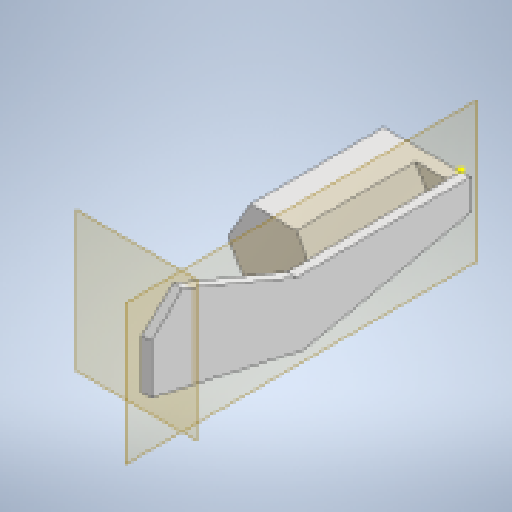
# Autodesk Inventor part: ArmSolenoidBoundingBoc
Saved by Autodesk Inventor 2023 (Build 270158000, 158)
## iProperties
Created: 2023-03-30
Part Number: ArmSolenoidBoundingBoc
Material: Generic
Document SubType Name: Modeling
Designer: LattePanda
Density: 1 g/cm^3
Appearance: Default
Author: LattePanda
Autodesk Inventor part; units mm, degrees
ref_plane "XZ Plane" through (0, 0, 0) normal (0, 1, 0) x (-1, 0, 0)
sketch "Sketch1" plane through (0, 0, 0) normal (1, 0, 0) x (0, 1, 0)
  line L0 (-24.1055, -88.5873) -> (-15.6118, -88.5873) construction
  line L1 (-20.9777, -35.0252) -> (-12.3846, 2.8126) construction
  line L2 (-11.1876, -82.4913) -> (-20.9871, -36.3884) construction
  line L3 (-10.1392, 12.7) -> (5.4091, 12.7)
  line L4 (5.4091, 12.7) -> (14.913, 2.8103)
  line L5 (14.913, 2.8103) -> (-0.1161, -33.4438)
  line L6 (-0.1161, -33.4438) -> (-0.1161, -88.5873)
  line L7 (-0.1161, -88.5873) -> (-9.8919, -88.5873)
  line L8 (-9.8919, -88.5873) -> (-21.1322, -35.7057)
  line L9 (-21.1322, -35.7057) -> (-10.1392, 12.7)
  line L10 (-0.1161, -27.3073) -> (-0.1161, -82.4913) construction
  arc A0 (9.8983, -7.957) -> (-12.3846, 2.8126) centre (0, 0) ccw construction
  point P0 (0, 0)
  constraints: 14 end point, 4 collinear, 3 tangent, 1 horizontal, 1 parallel
ref_plane "Work Plane1" through (3.048, -55.7199, -88.0008) normal (1, 0, 0) x (0, 0.7407454, 0.6717859)
extrude "Extrusion1" add sketch "Sketch1" along normal up to surface (3.048 mm away)
ref_plane "Work Plane2" through (86.0885, -0.1204, -88.5873) normal (0, 0, -1) x (0, -1, 0)
sketch "Sketch3" plane through (86.0885, -0.1204, -88.5873) normal (0, 0, -1) x (0, -1, 0)
  circle A0 centre (12.6956, 103.4693) radius 9.525 projected
  line L0 (12.6956, 89.0216) -> (0.1835, 96.2455)
  line L1 (0.1835, 96.2455) -> (0.1835, 110.6932)
  line L2 (0.1835, 110.6932) -> (12.6956, 117.9171)
  line L3 (12.6956, 117.9171) -> (25.2077, 110.6932)
  line L4 (25.2077, 110.6932) -> (25.2077, 96.2455)
  line L5 (25.2077, 96.2455) -> (12.6956, 89.0216)
  point P0 (-0.1204, 86.0885)
  constraints: 12 end point, 1 coincident, 13 other
ref_plane "Work Plane3" through (-20.1841, -15.6194, -46.4564) normal (0, 0, 1) x (0.8083839, 0.5886556, 0)
extrude "Extrusion2" add sketch "Sketch3" against normal up to surface (42.131 mm away) contours A0 | L0 L1 L2 L3 L4 L5
sketch "Sketch4" plane through (0, 0, 0) normal (-1, 0, 0) x (0, 0, 1)
  line L0 (-88.5873, -9.8919) -> (-88.5873, -0.1161) projected
  line L1 (-88.5873, -0.1161) -> (-33.4438, -0.1161) projected
  line L2 (-88.5873, -0.304) -> (-46.4564, -0.304) projected
  line L3 (-84.2988, -0.304) -> (-84.0662, -10.8529)
  line L4 (-35.7057, -21.1322) -> (-88.5873, -9.8919) projected
  point P0 (0, 0)
  constraints: 2 end point, 2 point on line
extrude "Extrusion3" add sketch "Sketch4" along normal blind 12.7
sketch "Sketch5" plane through (3.048, -0.1161, -88.5873) normal (0, 0, -1) x (-1, 0, 0)
  point P0 (3.048, 0.1161)
body "Solid1"
